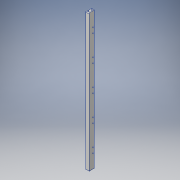
# Autodesk Inventor part: Winch_Plate_Rear
Saved by Autodesk Inventor 2016 (Build 200138000, 138)
## iProperties
Created: 2016-05-07
Part Number: Winch_Plate_Rear
Material: Aluminum 6061
Document SubType Name: Modeling
Designer: agmle
Density: 2.7 g/cm^3
Appearance: Aluminum - Flat
Mass: 319.883 g
Surface Area: 350.34 cm^2
Volume: 118.475 cm^3
Author: agmle
Autodesk Inventor part; units mm, degrees
note: some values were not read from the file. Chosen so that the rebuilt part matches the saved one: direction of "Hole1".
ref_plane "YZ Plane" through (0, 0, 0) normal (1, 0, 0) x (0, 1, 0)
ref_plane "XZ Plane" through (0, 0, 0) normal (0, 1, 0) x (-1, 0, 0)
ref_plane "XY Plane" through (0, 0, 0) normal (0, 0, 1) x (1, 0, 0)
sketch "Sketch1" plane through (0, 0, 0) normal (0, 1, 0) x (-1, 0, 0)
  line L0 (4.3175, 8.635) -> (-8.3825, 8.635)
  line L1 (-8.3825, 8.635) -> (-8.3825, -10.415)
  line L2 (-8.3825, -10.415) -> (4.3175, -10.415)
  line L3 (4.3175, -10.415) -> (4.3175, 8.635)
  point P0 (0, 0)
  dimension "d0" = 19.05
  dimension "d1" = 12.7
  constraints: 8 end point, 2 parallel, 1 horizontal, 1 perpendicular
  measures "d0" distance of L2.end L0.start
  measures "d1" distance of L0.start L0.end
extrude "Extrusion1" add sketch "Sketch1" along normal blind 504.952
sketch "Sketch2" plane through (8.3825, 0, 8.635) normal (1, 0, 0) x (0, 0, -1)
  line L0 (19.05, 0) -> (19.05, 504.952) projected
  line L1 (15.5575, 452.501) -> (15.5575, 433.451) construction
  line L2 (15.5575, 442.976) -> (19.05, 442.976) construction
  line L3 (15.5575, 357.251) -> (15.5575, 338.201) construction
  line L4 (15.5575, 347.726) -> (19.05, 347.726) construction
  line L5 (15.5575, 262.001) -> (15.5575, 242.951) construction
  line L6 (15.5575, 252.476) -> (19.05, 252.476) construction
  line L7 (15.5575, 166.751) -> (15.5575, 147.701) construction
  line L8 (15.5575, 157.226) -> (19.05, 157.226) construction
  line L9 (15.5575, 71.501) -> (15.5575, 52.451) construction
  line L10 (15.5575, 61.976) -> (19.05, 61.976) construction
  point P0 (8.635, 0)
  dimension "d4" = 19.05
  dimension "d5" = 3.4925
  dimension "d8" = 95.25
  constraints: 20 end point, 2 midpoint, 2 point on line, 2 vertical, 1 horizontal, 24 other
  measures "d4" distance of L1.end L1.start
  measures "d5" distance from line of L0 L1.start
  measures "d8" distance of L1.start L3.start
hole "Hole1" at (8.3825, 452.501, -6.9225) at (8.3825, 433.451, -6.9225) at (8.3825, 357.251, -6.9225) at (8.3825, 338.201, -6.9225) at (8.3825, 262.001, -6.9225) at (8.3825, 242.951, -6.9225) at (8.3825, 166.751, -6.9225) at (8.3825, 147.701, -6.9225) at (8.3825, 71.501, -6.9225) at (8.3825, 52.451, -6.9225) direction (-1, 0, 0) diameter 5.1054 end up to surface clearance for "Socket Head Cap Screw" size "#10" standard "Ansi Unified Screw Threads"
sketch "Sketch3" plane through (0, 504.952, 0) normal (0, 1, 0) x (1, 0, 0)
  circle A0 centre (3.9375, 5.97) radius 2.413 construction
  circle A1 centre (0.1275, -4.19) radius 2.413 construction
  line L0 (-4.3175, -8.635) -> (8.3825, -8.635) construction
  line L1 (-4.3175, 10.415) -> (-4.3175, -8.635) construction
  line L2 (8.3825, -8.635) -> (8.3825, 10.415) construction
  line L3 (8.3825, 10.415) -> (-4.3175, 10.415) construction
  point P0 (0, 0)
  dimension "d20" = 4.826
  dimension "d21" = 4.445
  dimension "d22" = 4.445
  dimension "d23" = 4.445
  dimension "d24" = 4.445
  constraints: 2 centre point, 2 coincident, 1 equal radius
  measures "d20" diameter of A0
  measures "d21" distance from line of L0 point (0.128, -4.19)
  measures "d22" distance from line of L1 point (0.128, -4.19)
  measures "d23" distance from line of L2 point (3.938, 5.97)
  measures "d24" distance from line of L3 point (3.938, 5.97)
hole "Hole2" at (0.1275, 504.952, 4.19) at (3.9375, 504.952, -5.97) direction (0, -1, 0) diameter 3.9624 depth 19.05 tip angle 118 thread size "10-32 UNF" class "2B" standard "ANSI Unified Screw Threads"
sketch "Sketch4" plane through (0, 0, 0) normal (0, -1, 0) x (1, 0, 0)
  line L0 (8.3825, -10.415) -> (-4.3175, -10.415) projected
  line L1 (-4.3175, -10.415) -> (-4.3175, 8.635) projected
  line L2 (8.3825, 8.635) -> (8.3825, -10.415) projected
  line L3 (-4.3175, 8.635) -> (8.3825, 8.635) projected
  point P0 (0, 0)
  point P1 (0.1275, -5.97)
  point P2 (3.9375, 4.19)
  dimension "d32" = 4.445
  dimension "d33" = 4.445
  dimension "d34" = 4.445
  dimension "d35" = 4.445
  measures "d32" distance from line of L0 point (0.128, -5.97)
  measures "d33" distance from line of L1 point (0.128, -5.97)
  measures "d34" distance from line of L2 point (3.938, 4.19)
  measures "d35" distance from line of L3 point (3.938, 4.19)
hole "Hole3" at (0.1275, 0, -5.97) at (3.9375, 0, 4.19) direction (0, 1, 0) diameter 3.9624 depth 19.05 tip angle 118 thread size "10-32 UNF" class "2B" standard "ANSI Unified Screw Threads"
fillet "Fillet1" radius 3.175 4 edges at (-4.3175, 504.952, -0.89) (8.3825, 0, -0.89) (2.0325, 0, 8.635) (2.0325, 504.952, 8.635)
equation "\"d22\" = d21"
equation "\"d23\" = d21"
equation "\"d24\" = d21"
equation "\"d32\" = d21"
equation "\"d33\" = d21"
equation "\"d34\" = d21"
equation "\"d35\" = d21"
body "Solid1"
